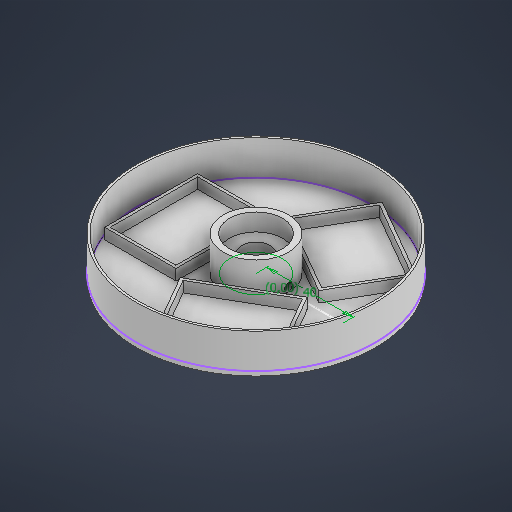
# Autodesk Inventor part: battery_spod
Saved by Autodesk Inventor 2027 (Build 310192060, 192F)
## iProperties
Created: 2026-05-17
Part Number: battery_spod
Material: Ogólny
Document SubType Name: Modeling
Designer: User
Density: 1 g/cm^3
Appearance: Domyślna
Author: User
Autodesk Inventor part; units mm, degrees
ref_plane "YZ Plane" through (0, 0, 0) normal (1, 0, 0) x (0, 1, 0)
ref_plane "XZ Plane" through (0, 0, 0) normal (0, 1, 0) x (-1, 0, 0)
ref_plane "XY Plane" through (0, 0, 0) normal (0, 0, 1) x (1, 0, 0)
sketch "Szkic1" plane through (0, 0, 0) normal (0, 1, 0) x (-1, 0, 0)
  circle A0 centre (0, 0) radius 54.26
  circle A1 centre (0, 0) radius 55.26
  dimension "d0" = 108.52
  dimension "d1" = 110.52
  constraints: 2 centre point, 2 coincident
  measures "d0" diameter of A0
  measures "d1" diameter of A1
extrude "Wyciągnięcie proste1" add sketch "Szkic1" along normal blind 2 contours A0 | A1
extrude "Wyciągnięcie proste2" add sketch "Szkic1" along normal blind 18
sketch "Szkic2" plane through (0, 2, 0) normal (0, 1, 0) x (1, 0, 0)
  circle A0 centre (-34.01, 19.66) radius 1.25
  circle A1 centre (0, 0) radius 54.26
  line L0 (-46.9152, 27.26) -> (46.9152, 27.26)
  line L1 (-34.01, 20.91) -> (-34.01, 27.26)
  line L2 (0, 27.26) -> (0, -54.26)
  circle A2 centre (0, 0) radius 54.26
  circle A3 centre (0, -39.24) radius 1.25
  circle A4 centre (34.01, 19.66) radius 1.25
  circle A5 centre (0, -39.24) radius 3
  circle A6 centre (34.01, 19.66) radius 3
  circle A7 centre (-34.01, 19.66) radius 3
  dimension "d6" = 2.5
  dimension "d7" = 6.35
  dimension "d8" = 27
  dimension "d9" = 34.01
  dimension "d10" = 2.5
  dimension "d11" = 66.5
  dimension "d12" = 39.24
  dimension "d13" = 7.6
  dimension "d14" = 6
  dimension "d15" = 6
  dimension "d16" = 6
  constraints: 7 centre point, 6 end point, 4 coincident, 3 point on circle, 2 point on line, 1 horizontal, 1 midpoint, 1 perpendicular, 1 symmetric about line, 1 vertical, 1 vertical alignment, 3 other
  measures "d7" distance of L1.start L1.end
  measures "d8" distance edge to line of A1 L0
  measures "d9" distance from line of A1.centre L1
  measures "d10" diameter of A3
  measures "d11" distance from line of L0 A3.centre
  measures "d12" distance of A1.centre A3.centre
  measures "d13" distance from line of point (-34.01, 19.66) L0
  measures "d14" diameter of A5
  measures "d15" diameter of A6
  measures "d16" diameter of A7
extrude "Wyciągnięcie proste3" [suppressed]
extrude "Wyciągnięcie proste4" [suppressed]
sketch "Szkic3" plane through (0, 2, 0) normal (0, 1, 0) x (1, 0, 0)
  circle A0 centre (0, 0) radius 12.2
  circle A1 centre (0, 0) radius 15
  circle A2 centre (0, 0) radius 6.5
  dimension "d21" = 24.4
  dimension "d22" = 30
  dimension "d25" = 13
  constraints: 3 centre point, 3 coincident
  measures "d21" diameter of A0
  measures "d22" diameter of A1
  measures "d25" diameter of A2
extrude "Wyciągnięcie proste5" add sketch "Szkic3" along normal up to surface (16 mm away) contours A1
extrude "Wyciągnięcie proste6" add sketch "Szkic3" along normal blind 8 contours A0
sketch "Szkic4" plane through (0, 2, 0) normal (0, 1, 0) x (1, 0, 0)
  circle A0 centre (0, 0) radius 6.5 projected
  line L0 (0, 0) -> (-32, 0)
  line L1 (0, 0) -> (32, 0) construction
  line L2 (-47.2, -20.2) -> (-16.8, -20.2)
  line L3 (-16.8, -20.2) -> (-16.8, 20.2)
  line L4 (-16.8, 20.2) -> (-47.2, 20.2)
  line L5 (-47.2, 20.2) -> (-47.2, -20.2)
  line L6 (-47.2, -20.2) -> (-16.8, 20.2) construction
  line L7 (-16.8, -20.2) -> (-47.2, 20.2) construction
  circle A1 centre (0, 0) radius 15
  circle A2 centre (0, 0) radius 54.26
  line L8 (-48.5, -21.5) -> (-15.5, -21.5)
  line L9 (-15.5, -21.5) -> (-15.5, 21.5)
  line L10 (-15.5, 21.5) -> (-48.5, 21.5)
  line L11 (-48.5, 21.5) -> (-48.5, -21.5)
  line L12 (-48.5, -21.5) -> (-15.5, 21.5) construction
  line L13 (-15.5, -21.5) -> (-48.5, 21.5) construction
  line L14 (0, 0) -> (16, -27.7128)
  circle A3 centre (0, 0) radius 54.26
  circle A4 centre (0, 0) radius 15
  line L15 (25.8937, -4.4492) -> (-9.0937, -24.6492)
  line L16 (26.3695, -2.6734) -> (-10.8695, -24.1734)
  line L17 (41.0937, -30.7764) -> (25.8937, -4.4492)
  line L18 (42.8695, -31.2522) -> (26.3695, -2.6734)
  line L19 (-9.0937, -24.6492) -> (6.1063, -50.9764)
  line L20 (-10.8695, -24.1734) -> (5.6305, -52.7522)
  line L21 (6.1063, -50.9764) -> (41.0937, -30.7764)
  line L22 (41.0937, -30.7764) -> (-9.0937, -24.6492) construction
  line L23 (42.8695, -31.2522) -> (-10.8695, -24.1734) construction
  line L24 (26.3695, -2.6734) -> (5.6305, -52.7522) construction
  line L25 (5.6305, -52.7522) -> (42.8695, -31.2522)
  line L26 (25.8937, -4.4492) -> (6.1063, -50.9764) construction
  line L27 (0, 0) -> (16, 27.7128)
  circle A5 centre (0, 0) radius 54.26
  circle A6 centre (0, 0) radius 15
  line L28 (-9.0937, 24.6492) -> (25.8937, 4.4492)
  line L29 (-10.8695, 24.1734) -> (26.3695, 2.6734)
  line L30 (6.1063, 50.9764) -> (-9.0937, 24.6492)
  line L31 (5.6305, 52.7522) -> (-10.8695, 24.1734)
  line L32 (25.8937, 4.4492) -> (41.0937, 30.7764)
  line L33 (26.3695, 2.6734) -> (42.8695, 31.2522)
  line L34 (41.0937, 30.7764) -> (6.1063, 50.9764)
  line L35 (6.1063, 50.9764) -> (25.8937, 4.4492) construction
  line L36 (5.6305, 52.7522) -> (26.3695, 2.6734) construction
  line L37 (-10.8695, 24.1734) -> (42.8695, 31.2522) construction
  line L38 (42.8695, 31.2522) -> (5.6305, 52.7522)
  line L39 (-9.0937, 24.6492) -> (41.0937, 30.7764) construction
  dimension "d28" = 32
  dimension "d29" = 180
  dimension "d30" = 30.4
  dimension "d31" = 40.4
  dimension "d32" = 33
  dimension "d33" = 43
  dimension "d36" = 360
  constraints: 80 end point, 8 coincident, 6 centre point, 4 horizontal, 4 midpoint, 4 parallel, 2 perpendicular, 1 collinear, 80 other
  measures "d28" distance of L0.start L0.end
  measures "d29" angle of L0 L1
  measures "d30" distance of L4.end L3.end
  measures "d31" distance of L3.end L2.end
  measures "d32" distance of L10.end L9.end
  measures "d33" distance of L9.end L8.end
extrude "Wyciągnięcie proste7" add sketch "Szkic4" along normal blind 5 contours L11 L10 L9 L8 | L18 L25 L20 L16 | L31 L38 L33 L29
move faces "Przesuń1" translate (0, -0.5, 0) faces at (-0.7683, 2, 2.0259)
sketch "Szkic5" plane through (0, 0, 0) normal (0, 0, 1) x (1, 0, 0)
  line L0 (26.3695, 2) -> (-10.8695, 2) projected
  line L1 (0, 2) -> (29.9975, 2.3855)
  line L2 (0, 2) -> (29.9975, 2)
  line L3 (29.9975, 2) -> (29.9975, 4)
  line L4 (29.9975, 4) -> (0, 4)
  line L5 (0, 4) -> (0, 2)
  point P0 (0, 0)
  dimension "d43" = 30
  dimension "d44" = 2
  constraints: 10 end point, 2 parallel, 1 horizontal, 1 perpendicular, 1 point on line
  measures "d43" distance of L1.start L1.end
  measures "d44" distance of L3.end L2.end
revolve "Obrót1" cut sketch "Szkic5" angle 360 about axis through (29.9975, 4, 0) along (-1, 0, 0) contours L5 L4 L3 L1
sketch "Szkic6" plane through (0, 2, 0) normal (0, 1, 0) x (1, 0, 0)
  circle A0 centre (0, 0) radius 54.26
  circle A1 centre (0, 0) radius 55.26
  line L0 (0, 0) -> (40, 0)
  line L1 (0, 0) -> (40, 0) construction
  dimension "d46" = 40
  dimension "d47" = 0
  constraints: 4 end point, 2 centre point, 2 coincident, 2 horizontal, 1 collinear
  measures "d46" distance of L0.start L0.end
  measures "d47" distance between parallel lines of L0 L1
